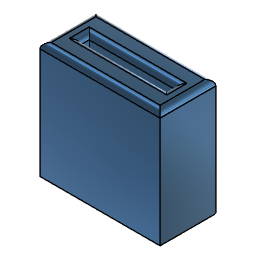
rasp berry pi 3 case (Autodesk Fusion 360 design; units mm, degrees)
Autodesk Fusion 360 part; units mm, degrees
sketch "Sketch1" plane through (0, 0, 0) normal (0, 0, 1) x (1, 0, 0)
  line L0 (53.75, -25) -> (-53.75, -25)
  line L1 (-53.75, -25) -> (-53.75, 25)
  line L2 (-53.75, 25) -> (53.75, 25)
  line L3 (53.75, 25) -> (53.75, -25)
  line L4 (53.75, -25) -> (-53.75, 25) construction
  line L5 (-53.75, -25) -> (53.75, 25) construction
  dimension "d4" = 107.5
  dimension "d5" = 50
  constraint horizontal L0
  constraint perpendicular L0 L1
  constraint parallel L0 L2
  constraint parallel L1 L3
  constraint coincident L4 origin
  constraint coincident L5 origin
  measures "d4" distance of L1.end L2.end
  measures "d5" distance of L0.end L1.end
extrude "Extrude1" add sketch "Sketch1" along normal blind 104
sketch "Sketch2" plane through (0, 0, 104) normal (0, 0, 1) x (-1, 0, 0)
  line L0 (-53.75, -25) -> (53.75, -25)
  line L1 (53.75, -25) -> (53.75, 25)
  line L2 (53.75, 25) -> (-53.75, 25)
  line L3 (-53.75, 25) -> (-53.75, -25)
  line L4 (-38.75, 4) -> (38.75, 4)
  line L5 (38.75, 4) -> (38.75, -4)
  line L6 (38.75, -4) -> (-38.75, -4)
  line L7 (-38.75, -4) -> (-38.75, 4)
  line L8 (-38.75, 4) -> (38.75, -4) construction
  line L9 (38.75, 4) -> (-38.75, -4) construction
  dimension "d8" = 77.5
  dimension "d9" = 8
  constraint horizontal L4
  constraint perpendicular L4 L5
  constraint parallel L4 L6
  constraint parallel L5 L7
  constraint coincident L8 origin
  constraint coincident L9 origin
  measures "d8" distance of L5.end L6.end
  measures "d9" distance of L4.end L5.end
extrude "Extrude2" cut sketch "Sketch2" against normal blind 94 contours L4 L5 L6 L7
fillet "Fillet1" radius 5 1 faces at (12.9167, -18, 104)
equation "bredde = 77.5 mm"
equation "høyde = 312 mm"
equation "tykkelse = 8 mm"
equation "d4 = bredde + 30 mm"
equation "d6 = høyde / 3"
equation "d8 = bredde"
equation "d9 = tykkelse"
equation "d10 = -høyde / 3 + 10 mm"
